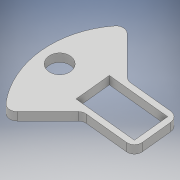
# Autodesk Inventor part: ir-holder
Saved by Autodesk Inventor 2018 (Build 220112000, 112)
## iProperties
Created: 2018-03-21
Part Number: ir-holder
Material: Generic
Document SubType Name: Modeling
Designer: Matt
Density: 1 g/cm^3
Appearance: Default
Author: Matt
Autodesk Inventor part; units mm, degrees
ref_plane "YZ Plane" through (0, 0, 0) normal (1, 0, 0) x (0, 1, 0)
ref_plane "XZ Plane" through (0, 0, 0) normal (0, 1, 0) x (-1, 0, 0)
ref_plane "XY Plane" through (0, 0, 0) normal (0, 0, 1) x (1, 0, 0)
sketch "Sketch1" plane through (0, 0, 0) normal (0, 0, 1) x (1, 0, 0)
  arc A0 (-2.2, 21.8897) -> (-21.8897, 2.2) centre (0, 0) ccw
  line L0 (-11.05, 0) -> (-19.8997, 0)
  line L1 (0, 11.05) -> (0, 19.8997)
  line L2 (0, 0) -> (22, 0) construction
  circle A1 centre (-12.1976, 12.1976) radius 2.8
  line L3 (0.5858, 7.4045) -> (6.9261, 1.0642)
  arc A2 (-21.8897, 2.2) -> (-19.8997, 0) centre (-19.8997, 2) ccw
  arc A3 (0, 19.8997) -> (-2.2, 21.8897) centre (-2, 19.8997) ccw
  line L4 (-8.5302, 2.5198) -> (-9.2373, 3.2269)
  line L5 (-3.2269, 9.2373) -> (-2.5198, 8.5302)
  line L6 (-0.1156, -5.8948) -> (-8.5302, 2.5198)
  line L7 (-2.5198, 8.5302) -> (5.8948, 0.1156)
  line L8 (-11.05, 0) -> (-8.8187, 0)
  line L9 (-7.4045, -0.5858) -> (-1.0642, -6.9261)
  line L10 (0, 11.05) -> (0, 8.8187)
  arc A4 (-7.4045, -0.5858) -> (-8.8187, 0) centre (-8.8187, -2) ccw
  arc A5 (0, 8.8187) -> (0.5858, 7.4045) centre (2, 8.8187) ccw
  arc A6 (0, 11.05) -> (-1.5191, 10.9451) centre (0, 0) ccw
  line L11 (5.8948, 0.1156) -> (7.309, -1.2986)
  line L12 (-0.1156, -5.8948) -> (1.2986, -7.309)
  line L13 (-0.1156, -5.8948) -> (1.8844, -5.8948) construction
  line L14 (1.2986, -7.309) -> (7.309, -1.2986)
  line L15 (-9.2373, 3.2269) -> (-3.2269, 9.2373)
  line L16 (-1.0642, -6.9261) -> (-0.1156, -7.8747)
  line L17 (2.7128, -7.8747) -> (7.8747, -2.7128)
  line L18 (7.8747, 0.1156) -> (6.9261, 1.0642)
  arc A7 (-10.2177, 4.2073) -> (-10.7101, 2.7198) centre (0, 0) ccw
  arc A8 (-10.9451, 1.5191) -> (-11.05, 0) centre (0, 0) ccw
  arc A9 (7.8747, -2.7128) -> (7.8747, 0.1156) centre (6.4605, -1.2986) ccw
  arc A10 (-0.1156, -7.8747) -> (2.7128, -7.8747) centre (1.2986, -6.4605) ccw
  point P0 (-22, 0)
  point P1 (0, 22)
  point P2 (0, 7.9903)
  point P3 (-4.2073, 10.2177)
  dimension "d1" = 44
  dimension "d3" = 5.6
  dimension "d4" = 17.25
  dimension "d6" = 15.6271
  dimension "d16" = 1
  dimension "d18" = 2
  dimension "d19" = 1
  dimension "d20" = 2
  dimension "d21" = 2
  dimension "d22" = 45
  dimension "d23" = 14.9
  dimension "d24" = 2
  constraints: 38 end point, 22 point on circle, 12 tangent, 11 centre point, 9 point on line, 4 horizontal, 4 perpendicular, 2 coincident, 2 equal radius, 1 equal length, 1 parallel, 1 vertical
  measures "d1" diameter of A0
  measures "d3" diameter of A1
  measures "d4" distance of point (0, 0) A1.centre
  measures "d6" distance of L1.start L0.start
  measures "d16" distance of L4.start L4.end
  measures "d18" radius of A4
  measures "d19" distance of L5.start L5.end
  measures "d20" distance of L7.end L11.end
  measures "d21" distance of L6.start L12.end
  measures "d22" angle of L12 L13
  measures "d23" distance between parallel lines of L14 L15
  measures "d24" radius of A9
extrude "Extrusion1" add sketch "Sketch1" along normal blind 2.4
body "Solid1"
